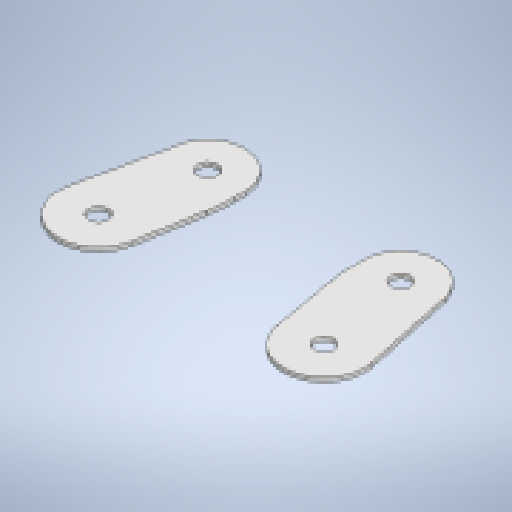
# Autodesk Inventor part: IntakeHolder
Saved by Autodesk Inventor 2023 (Build 270158000, 158)
## iProperties
Created: 2022-09-11
Part Number: IntakeHolder
Material: Generic
Document SubType Name: Modeling
Designer: deli
Density: 1 g/cm^3
Appearance: Default
Author: deli
Autodesk Inventor part; units mm, degrees
ref_plane "YZ Plane" through (0, 0, 0) normal (1, 0, 0) x (0, 1, 0)
ref_plane "XZ Plane" through (0, 0, 0) normal (0, 1, 0) x (-1, 0, 0)
ref_plane "XY Plane" through (0, 0, 0) normal (0, 0, 1) x (1, 0, 0)
sketch "Sketch1" plane through (0, 0, 0) normal (0, 1, 0) x (-1, 0, 0)
  circle A0 centre (19.4316, 162.4913) radius 7
  circle A1 centre (19.4316, 162.4913) radius 24 construction
  circle A2 centre (7.7103, 228.9658) radius 24 construction
  circle A3 centre (7.7103, 228.9658) radius 7
  circle A4 centre (157.4316, 162.4913) radius 7
  circle A5 centre (169.1528, 228.9658) radius 7
  circle A6 centre (169.1528, 228.9658) radius 24 construction
  circle A7 centre (157.4316, 162.4913) radius 24 construction
  line L0 (157.4316, 162.4913) -> (19.4316, 162.4913) construction
  line L1 (7.7103, 228.9658) -> (19.4316, 162.4913) construction
  line L2 (169.1528, 228.9658) -> (157.4316, 162.4913) construction
  circle A8 centre (88.4316, 133.6115) radius 50.8 construction
  line L3 (36.2697, 234.0016) -> (44.4123, 187.8226)
  line L4 (140.5934, 234.0016) -> (132.4508, 187.8226)
  arc A9 (36.2697, 234.0016) -> (-20.643, 222.8757) centre (7.7103, 228.9658) ccw
  arc A10 (197.5061, 222.8757) -> (140.5934, 234.0016) centre (169.1528, 228.9658) ccw
  arc A11 (-6.4775, 156.9262) -> (45.9316, 162.4913) centre (19.4316, 162.4913) ccw
  arc A12 (130.9316, 162.4913) -> (183.3406, 156.9262) centre (157.4316, 162.4913) ccw
  line L5 (197.5061, 222.8757) -> (183.3406, 156.9262)
  line L6 (-20.643, 222.8757) -> (-6.4775, 156.9262)
  line L7 (45.9316, 162.4913) -> (45.9316, 170.4578)
  line L8 (130.9316, 162.4913) -> (130.9316, 170.4578)
  arc A13 (45.9316, 170.4578) -> (44.4123, 187.8226) centre (-54.0684, 170.4578) ccw
  arc A14 (132.4508, 187.8226) -> (130.9316, 170.4578) centre (230.9316, 170.4578) ccw
  point P0 (0, 0)
  dimension "d0" = 14
  dimension "d1" = 48
  dimension "d2" = 48
  dimension "d3" = 14
  dimension "d4" = 67.5
  dimension "d5" = 48
  dimension "d6" = 14
  dimension "d7" = 14
  dimension "d8" = 48
  dimension "d9" = 67.5
  dimension "d10" = 90
  dimension "d11" = 100
  dimension "d12" = 100
  dimension "d13" = 101.6
  dimension "d18" = 5
  dimension "d19" = 5
  dimension "d21" = 85
  dimension "d22" = 100
  dimension "d23" = 100
  constraints: 18 end point, 15 centre point, 14 tangent, 12 point on circle, 8 coincident, 2 parallel, 2 vertical, 1 equal radius, 1 horizontal, 1 point on line
  measures "d0" diameter of A0
  measures "d1" diameter of A1
  measures "d2" diameter of A2
  measures "d3" diameter of A3
  measures "d4" distance of A0.centre L1.start
  measures "d5" diameter of A6
  measures "d6" diameter of A5
  measures "d7" diameter of A4
  measures "d8" diameter of A7
  measures "d9" distance of A4.centre A5.centre
  measures "d11" angle of L0 L2
  measures "d12" angle of L0 L1
  measures "d13" diameter of A8
  measures "d18" distance edge to line of A2 L3
  measures "d19" distance edge to line of A6 L4
  measures "d21" distance between parallel lines of L8 L7
  measures "d22" radius of A13
  measures "d23" radius of A14
extrude "Extrusion1" add sketch "Sketch1" along normal blind 3.175
equation "\"d2\" = d1"
equation "\"d3\" = d0"
equation "\"d5\" = d1"
equation "\"d6\" = d0"
equation "\"d7\" = d0"
equation "\"d8\" = d1"
equation "\"d9\" = d4"
equation "\"d12\" = d11"
equation "\"d19\" = d18"
equation "\"d23\" = d22"
equation "\"d17\" = d16"
equation "\"d16\" = 5"
body "Solid1"
